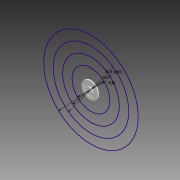
# Autodesk Inventor part: Base
Saved by Autodesk Inventor 2020 (Build 240168000, 168)
## iProperties
Created: 2021-03-19
Part Number: Base
Material: Generic
Document SubType Name: Modeling
Designer: DDeGo
Density: 1 g/cm^3
Appearance: Default
Author: DDeGo
Autodesk Inventor part; units mm, degrees
ref_plane "YZ Plane" through (0, 0, 0) normal (1, 0, 0) x (0, 1, 0)
ref_plane "XZ Plane" through (0, 0, 0) normal (0, 1, 0) x (-1, 0, 0)
ref_plane "XY Plane" through (0, 0, 0) normal (0, 0, 1) x (1, 0, 0)
sketch "Sketch1" plane through (0, 0, 0) normal (0, 0, 1) x (1, 0, 0)
  circle A0 centre (0, 0) radius 87.5
  dimension "d0" = 175
  constraints: 1 centre point, 1 coincident
  measures "d0" diameter of A0
extrude "Extrusion1" add sketch "Sketch1" along normal blind 5
sketch "Sketch2" plane through (0, 0, 0) normal (0, 0, -1) x (-1, 0, 0)
  circle A0 centre (0, 0) radius 200
  circle A1 centre (0, 0) radius 300
  circle A2 centre (0, 0) radius 400
  circle A3 centre (0, 0) radius 500
  dimension "d3" = 400
  dimension "d4" = 600
  dimension "d5" = 800
  dimension "d6" = 1000
  constraints: 4 centre point, 4 coincident
  measures "d3" diameter of A0
  measures "d4" diameter of A1
  measures "d5" diameter of A2
  measures "d6" diameter of A3
sketch "Sketch3" plane through (0, 0, 0) normal (1, 0, 0) x (0, 1, 0)
  line L0 (87.5, 5) -> (-87.5, 5) projected
  line L1 (0, 5) -> (0, 48.7563) construction
  line L2 (87.5, 5) -> (87.5, 11)
  line L3 (87.5, 11) -> (50, 11)
  line L4 (50, 11) -> (50, 7)
  line L5 (50, 7) -> (33.5, 7)
  line L6 (33.5, 7) -> (33.5, 11)
  line L7 (25, 12.5) -> (25, 17.5)
  line L8 (25, 17.5) -> (0, 17.5)
  line L9 (0, 17.5) -> (0, 5)
  line L10 (0, 5) -> (87.5, 5)
  line L11 (25, 12.5) -> (26.5, 12.5)
  line L12 (26.5, 12.5) -> (26.5, 11)
  line L13 (26.5, 11) -> (33.5, 11)
  point P0 (0, 0)
  dimension "d8" = 6
  dimension "d9" = 2
  dimension "d15" = 33.5
  dimension "d32" = 12.5
  dimension "d33" = 25
  dimension "d36" = 1.5
  dimension "d37" = 50
  dimension "d38" = 5.5
  dimension "d39" = 4
  constraints: 26 end point, 8 perpendicular, 3 vertical, 1 collinear, 1 horizontal, 1 midpoint, 1 point on line
  measures "d8" distance between parallel lines of L0 L3
  measures "d9" distance between parallel lines of L0 L5
  measures "d15" distance between parallel lines of L1 L6
  measures "d32" distance between parallel lines of L8 L0
  measures "d33" distance between parallel lines of L1 L7
  measures "d36" distance of L7.start L11.end
  measures "d37" distance between parallel lines of L4 L9
  measures "d38" distance between parallel lines of L11 L5
  measures "d39" distance between parallel lines of L5 L13
revolve "Revolution1" add sketch "Sketch3" angle 360 about axis through (0, 0, 5) along (0, 0, 1)
sketch "Sketch4" plane through (0, 0, 17.5) normal (0, 0, 1) x (1, 0, 0)
  line L0 (0, 0) -> (-20, 0) construction
  circle A0 centre (-20, 0) radius 2.75
  circle A1 centre (-14.1421, -14.1421) radius 2.75
  circle A2 centre (0, -20) radius 2.75
  circle A3 centre (14.1421, -14.1421) radius 2.75
  circle A4 centre (20, 0) radius 2.75
  circle A5 centre (14.1421, 14.1421) radius 2.75
  circle A6 centre (0, 20) radius 2.75
  circle A7 centre (-14.1421, 14.1421) radius 2.75
  dimension "d16" = 20
  dimension "d17" = 5.5
  dimension "d20" = 360
  constraints: 9 coincident, 8 centre point, 2 end point, 1 horizontal, 25 other
  measures "d16" distance of L0.start L0.end
  measures "d17" diameter of A0
extrude "Extrusion2" cut sketch "Sketch4" against normal through all
sketch "Sketch5" plane through (0, 0, 0) normal (0, 0, -1) x (-1, 0, 0)
  circle A0 centre (-14.1421, 14.1421) radius 2.75 construction
  circle A1 centre (-14.1421, 14.1421) radius 4.75
  circle A2 centre (-20, 0) radius 4.75
  circle A3 centre (-14.1421, -14.1421) radius 4.75
  circle A4 centre (0, -20) radius 4.75
  circle A5 centre (14.1421, -14.1421) radius 4.75
  circle A6 centre (20, 0) radius 4.75
  circle A7 centre (14.1421, 14.1421) radius 4.75
  circle A8 centre (0, 20) radius 4.75
  point P0 (0, 0)
  point P1 (-19.5123, 15.6291)
  point P2 (-15.6291, 19.5123)
  dimension "d24" = 9.5
  dimension "d27" = 360
  constraints: 8 centre point, 1 coincident, 18 other
  measures "d24" diameter of A1
extrude "Extrusion3" cut sketch "Sketch5" against normal blind 6
body "Solid1"
